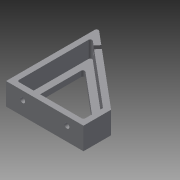
# Autodesk Inventor part: oled_halterung_W162_links
Saved by Autodesk Inventor 2015 (Build 190159000, 159)
## iProperties
Created: 2014-11-18
Part Number: oled_halterung_W162_links
Material: Generisch
Document SubType Name: Modeling
Designer: Zephram
Density: 1 g/cm^3
Appearance: Vorgabe
Author: Zephram
Autodesk Inventor part; units mm, degrees
ref_plane "YZ Plane" through (0, 0, 0) normal (1, 0, 0) x (0, 1, 0)
ref_plane "XZ Plane" through (0, 0, 0) normal (0, 1, 0) x (-1, 0, 0)
ref_plane "XY Plane" through (0, 0, 0) normal (0, 0, 1) x (1, 0, 0)
sketch "Skizze1" plane through (0, 0, 0) normal (0, 0, 1) x (1, 0, 0)
  line L0 (0, 0) -> (0, 50.2422)
  line L1 (0, 50.2422) -> (42, 15)
  line L2 (42, 15) -> (42, 0)
  line L3 (42, 0) -> (0, 0)
  line L4 (6.5, 36.3029) -> (6.5, 6.5)
  line L5 (6.5, 6.5) -> (35.5, 6.5)
  line L6 (35.5, 6.5) -> (35.5, 11.969)
  line L7 (35.5, 11.969) -> (6.5, 36.3029)
  dimension "d0" = 130
  dimension "d1" = 15
  dimension "d2" = 42
  dimension "d3" = 6.5
  dimension "d4" = 6.5
  dimension "d5" = 6.5
  dimension "d6" = 6.5
  constraints: 16 end point, 5 parallel, 1 perpendicular, 1 vertical
  measures "d0" angle of L2 L1
  measures "d1" distance of L1.end L2.end
  measures "d2" distance of L2.end L0.start
  measures "d3" distance between parallel lines of L3 L5
  measures "d4" distance between parallel lines of L0 L4
  measures "d5" distance between parallel lines of L1 L7
  measures "d6" distance between parallel lines of L2 L6
extrude "Extrusion1" add sketch "Skizze1" along normal blind 12
sketch "Skizze2" plane through (0, 0, 12) normal (0, 0, 1) x (1, 0, 0)
  line L0 (3, 43.8087) -> (3, 3)
  line L1 (3, 3) -> (39, 3)
  line L2 (39, 3) -> (39, 13.6011)
  line L3 (39, 13.6011) -> (3, 43.8087)
  line L4 (0, 0) -> (42, 0) projected
  line L5 (0, 50.2422) -> (0, 0) projected
  line L6 (42, 15) -> (0, 50.2422) projected
  line L7 (42, 0) -> (42, 15) projected
  dimension "d9" = 3
  dimension "d10" = 3
  dimension "d11" = 3
  dimension "d12" = 3
  constraints: 8 end point, 4 parallel, 1 horizontal, 1 perpendicular
  measures "d9" distance between parallel lines of L6 L3
  measures "d10" distance between parallel lines of L5 L0
  measures "d11" distance between parallel lines of L4 L1
  measures "d12" distance between parallel lines of L7 L2
extrude "Extrusion2" cut sketch "Skizze2" against normal blind 9 contours L3 L2 L1 L0
sketch "Skizze3" plane through (3, 3, 12) normal (0, 1, 0) x (1, 0, 0)
  line L0 (-3, 0) -> (-3, 12) projected
  line L1 (-3, 12) -> (39, 12) projected
  line L2 (39, 12) -> (39, 0) projected
  line L3 (39, 0) -> (36, 0) projected
  line L4 (36, 0) -> (0, 0) projected
  line L5 (0, 0) -> (-3, 0) projected
  line L6 (36, 0) -> (36, 9) projected
  line L7 (36, 9) -> (0, 9) projected
  line L8 (0, 9) -> (0, 0) projected
  line L9 (0, 0) -> (0, 9) projected
  line L10 (36, 0) -> (36, 9) projected
  line L11 (36, 4.5) -> (0, 4.5)
  point P0 (6, 4.5)
  point P1 (30, 4.5)
  dimension "d15" = 6
  dimension "d17" = 6
  constraints: 2 end point, 2 midpoint, 2 point on line
  measures "d15" distance of point (6, 4.5) L11.end
  measures "d17" distance of point (30, 4.5) L11.start
hole "Bohrung1" at (9, 3, 7.5) at (33, 3, 7.5) direction (0, -1, 0) diameter 2.7 depth 8 tip angle 118
fillet "Rundung1" radius 1 8 edges at (39, 13.6011, 7.5) (35.5, 11.969, 1.5) (3, 43.8087, 7.5) (6.5, 36.3029, 1.5) (6.5, 6.5, 1.5) (3, 3, 7.5) (35.5, 6.5, 1.5) (39, 3, 7.5)
sketch "Skizze4" plane through (4.6428, 42.4302, 3) normal (-0.6427876, -0.7660444, 0) x (0.7660444, -0.6427876, 0)
  line L0 (0, 9) -> (44.3838, 9) projected
  line L1 (44.3838, 9) -> (44.3838, 0) projected
  line L2 (0, 0) -> (0, 9) projected
  point P0 (23.717, -3)
  point P1 (40.3838, 5)
  point P2 (4.3838, 6.5)
  dimension "d26" = 4
  dimension "d27" = 4
  dimension "d28" = 2.5
  dimension "d29" = 40
  dimension "d30" = 4.3838
  measures "d26" distance from line of L0 point (40.384, 5)
  measures "d27" distance from line of L1 point (40.384, 5)
  measures "d28" distance from line of L0 point (4.384, 6.5)
  measures "d29" distance from line of L1 point (4.384, 6.5)
  measures "d30" distance from line of point (4.384, 6.5) L2
hole "Bohrung2" at (35.5786, 16.472, 8) at (8.001, 39.6123, 9.5) direction (0.6427876, 0.7660444, 0) diameter 2.5 depth 8 tip angle 118
sketch "Skizze5" plane through (4.6428, 42.4302, 3) normal (-0.6427876, -0.7660444, 0) x (0.7660444, -0.6427876, 0)
  circle A0 centre (4.3838, 6.5) radius 1.25 projected
  line L0 (46.2491, 9) -> (-8.578, 9) projected
  line L1 (3.1338, 6.5) -> (3.1338, 9)
  line L2 (5.6338, 9) -> (5.6338, 6.5)
  point P0 (23.717, -3)
  constraints: 4 end point, 2 point on circle, 2 point on line, 1 perpendicular, 1 tangent
extrude "Extrusion3" cut sketch "Skizze5" against normal blind 15.25 contours A0 L1 L0 L2
sketch "Mutter im Winkel" plane through (0, 0, 12) normal (0, 0, 1) x (1, 0, 0)
  line L0 (0, 50.2422) -> (42, 15) projected
  line L1 (9.9294, 41.9105) -> (4.53, 35.4757)
  line L2 (7.0435, 40.4158) -> (8.9718, 42.7139) projected
  line L3 (8.9586, 38.8088) -> (7.0435, 40.4158) projected
  line L4 (10.2991, 37.684) -> (5.7029, 41.5407)
  line L5 (5.7029, 41.5407) -> (5.3815, 41.1577)
  line L6 (5.3815, 41.1577) -> (9.9777, 37.3009)
  line L7 (9.9777, 37.3009) -> (10.2991, 37.684)
  line L8 (4.6428, 42.4302) -> (38.6428, 13.9008) projected
  line L9 (9.7671, 37.4777) -> (8.4815, 35.9456)
  line L10 (8.4815, 35.9456) -> (4.3066, 39.4488)
  line L11 (4.3066, 39.4488) -> (5.5921, 40.9809)
  point P0 (0, 0)
  dimension "d40" = 1.25
  dimension "d41" = 5.4
  dimension "d43" = 0.5
  dimension "d44" = 6
  dimension "d45" = 5.45
  dimension "d46" = 2
  constraints: 16 end point, 4 perpendicular, 4 point on line, 3 parallel, 2 other
  measures "d40" distance between parallel lines of L2 L1
  measures "d41" distance from line of L1.end L3
  measures "d43" distance from line of L6.end L4
  measures "d44" distance between parallel lines of L5 L7
  measures "d45" distance between parallel lines of L11 L9
  measures "d46" distance between parallel lines of L6 L10
fillet "Rundung2" radius 1 1 edges at (0, 50.2422, 6)
